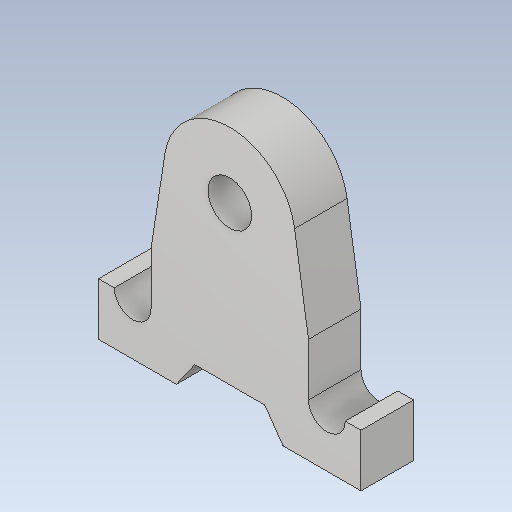
# Autodesk Inventor part: 新型４留め具
Saved by Autodesk Inventor 2020 (Build 240168000, 168)
## iProperties
Created: 2019-06-10
Part Number: 新型４留め具
Material: アルミニウム 2014-T4
Document SubType Name: Modeling
Designer: tanjihayato
Density: 2.8 g/cm^3
Appearance: サテン
Mass: 0.970113 g
Surface Area: 4.28118 cm^2
Volume: 0.346469 cm^3
Author: tanjihayato
Autodesk Inventor part; units mm, degrees
ref_plane "YZ Plane" through (0, 0, 0) normal (1, 0, 0) x (0, 1, 0)
ref_plane "XZ Plane" through (0, 0, 0) normal (0, 1, 0) x (-1, 0, 0)
ref_plane "XY Plane" through (0, 0, 0) normal (0, 0, 1) x (1, 0, 0)
sketch "スケッチ1" plane through (0, 0, 0) normal (0, 0, 1) x (1, 0, 0)
  circle A0 centre (0, 0) radius 1.25
  circle A1 centre (0, 0) radius 3.75
  line L0 (-7.5, -10.5) -> (7.5, -10.5)
  line L1 (7.5, -10.5) -> (7.5, -7.5)
  line L2 (7.5, -7.5) -> (4.5, -7.5)
  line L3 (4.5, -7.5) -> (4.5, -4.5)
  line L4 (-7.5, -10.5) -> (-7.5, -7.5)
  line L5 (-7.5, -7.5) -> (-4.5, -7.5)
  line L6 (-4.5, -7.5) -> (-4.5, -4.5)
  line L7 (-4.5, -4.5) -> (-3.7049, 0.5799)
  line L8 (3.7049, 0.5799) -> (4.5, -4.5)
  arc A2 (-6.6, -7.5) -> (-4.5, -7.5) centre (-5.55, -7.5) ccw
  arc A3 (4.5, -7.5) -> (6.6, -7.5) centre (5.55, -7.5) ccw
  dimension "d0" = 2.5
  dimension "d1" = 7.5
  dimension "d2" = 15
  dimension "d3" = 3
  dimension "d4" = 3
  dimension "d5" = 3
  dimension "d6" = 3
  dimension "d7" = 3
  dimension "d8" = 3
  dimension "d9" = 4.5
  dimension "d10" = 7.5
  dimension "d11" = 2.1
  dimension "d12" = 2.1
  constraints: 18 end point, 6 point on circle, 5 perpendicular, 4 centre point, 4 point on line, 4 tangent, 2 coincident, 1 horizontal, 1 vertical
  measures "d0" diameter of A0
  measures "d1" diameter of A1
  measures "d2" distance of L0.start L0.end
  measures "d3" distance of L0.end L1.end
  measures "d4" distance of L1.end L2.end
  measures "d5" distance of L2.end L3.end
  measures "d6" distance of L0.start L4.end
  measures "d7" distance of L4.end L5.end
  measures "d8" distance of L5.end L6.end
  measures "d9" distance from line of A0.centre L3
  measures "d10" distance from line of point (0, 0) L2
  measures "d11" diameter of A2
  measures "d12" diameter of A3
extrude "押し出し1" add sketch "スケッチ1" along normal blind 3 contours A1 | A1 L8 L3 A3 L2 L1 L0 L4 L5 A2 L6 L7
sketch "スケッチ2" plane through (0, 0, 3) normal (0, 0, 1) x (1, 0, 0)
  circle A0 centre (0, 0) radius 1.25 projected
  arc A1 (3.7049, 0.5799) -> (-3.7049, 0.5799) centre (0, 0) ccw projected
  line L0 (-3.7049, 0.5799) -> (-4.5, -4.5) projected
  line L1 (-4.5, -4.5) -> (-4.5, -7.5) projected
  arc A2 (-6.6, -7.5) -> (-4.5, -7.5) centre (-5.55, -7.5) ccw projected
  line L2 (-6.6, -7.5) -> (-7.5, -7.5) projected
  line L3 (-7.5, -7.5) -> (-7.5, -10.5) projected
  line L4 (-7.5, -10.5) -> (7.5, -10.5) projected
  line L5 (7.5, -10.5) -> (7.5, -7.5) projected
  line L6 (7.5, -7.5) -> (6.6, -7.5) projected
  arc A3 (4.5, -7.5) -> (6.6, -7.5) centre (5.55, -7.5) ccw projected
  line L7 (4.5, -7.5) -> (4.5, -4.5) projected
  line L8 (4.5, -4.5) -> (3.7049, 0.5799) projected
  line L9 (-3.0503, -10.5) -> (-2, -9)
  line L10 (-2, -9) -> (2, -9)
  line L11 (2, -9) -> (3.0503, -10.5)
  dimension "d15" = 125
  dimension "d16" = 125
  dimension "d17" = 4
  dimension "d18" = 2
  dimension "d19" = 1.5
  constraints: 6 end point, 2 point on line, 1 horizontal
  measures "d15" angle of L4 L11
  measures "d16" angle of L4 L9
  measures "d17" distance of L9.end L10.end
  measures "d18" horizontal distance of L10.end point (0, 0)
  measures "d19" distance between parallel lines of L4 L10
extrude "押し出し2" cut sketch "スケッチ2" against normal blind 3 contours L4 L9 L10 L11
